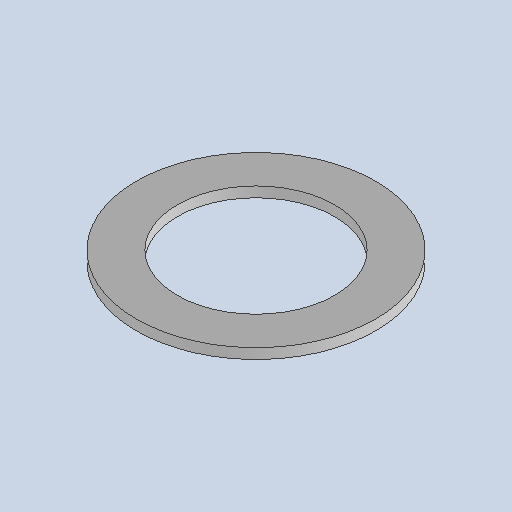
# Autodesk Inventor part: PRS 9432 FDS free flange DN90_1200
Saved by Autodesk Inventor 2026.2 (Build 302298000, 298)
## iProperties
Created: 2025-02-13
Part Number: PRS 9432 FDS free flange DN90_1200
Material: Steel
Document SubType Name: Sheet Metal
Designer: admin
Mass: 665.861 g
Surface Area: 279.916 cm^2
Volume: 84.823 cm^3
Density: 7.85 g/cm^3
Flat Pattern Width: 14 cm
Flat Pattern Length: 14 cm
Flat Pattern Area: 196 cm^2
Sheet Metal Rule: AISI304 4mm Die 32
Sheet Metal Width: 140,000 mm
Sheet Metal Length: 140,000 mm
Sheet Metal Area: 19600,000 mm^2
Appearance: Default
Author: pokla
Autodesk Inventor part; units mm, degrees
ref_plane "YZ Plane" through (0, 0, 0) normal (1, 0, 0) x (0, 1, 0)
ref_plane "XZ Plane" through (0, 0, 0) normal (0, 1, 0) x (-1, 0, 0)
ref_plane "XY Plane" through (0, 0, 0) normal (0, 0, 1) x (1, 0, 0)
sketch "Sketch2" plane through (0, 0, 0) normal (0, 0, 1) x (1, 0, 0)
  circle A0 centre (0, 0) radius 46
  circle A1 centre (0, 0) radius 70
  dimension "d25" = 92
  dimension "d27" = 140
  measures "d25" diameter of A0
  measures "d27" diameter of A1
extrude "Plate2" add sketch "Sketch2" along normal blind 6
equation "\"d14\" = Thickness"
equation "\"BendReliefWidth\" = Thickness"
equation "\"BendReliefDepth\" = 0.5 * Thickness"
equation "\"CornerReliefSize\" = 4 * Thickness"
equation "\"MinimumRemnant\" = 2 * Thickness"
equation "\"TransitionRadius\" = BendRadius"
equation "\"JacobiRadiusSize\" = BendRadius"
equation "\"GapSize\" = Thickness"
equation "\"Thickness\" = 6"
equation "\"BendRadius\" = 6"
body "Solid3"
